Autodesk Inventor part; units mm, degrees
(part 2 of 2)
  line L213 (3.5687, 9.8336) -> (2.9549, 9.8336)
  arc A527 (2.9549, 9.8526) -> (2.9549, 9.8145) centre (2.9549, 9.8336) ccw
  arc A528 (3.5687, 9.8145) -> (3.5687, 9.8526) centre (3.5687, 9.8336) ccw
  arc A529 (2.8321, 9.9563) -> (2.9549, 9.8336) centre (2.9549, 9.9564) ccw
  arc A530 (2.8512, 9.9563) -> (2.8131, 9.9563) centre (2.8321, 9.9563) ccw
  arc A531 (2.9549, 9.8145) -> (2.9549, 9.8526) centre (2.9549, 9.8336) ccw
  line L214 (2.8321, 9.9563) -> (2.8321, 9.9972)
  arc A532 (2.8512, 9.9972) -> (2.8131, 9.9972) centre (2.8321, 9.9972) ccw
  arc A533 (2.8131, 9.9563) -> (2.8512, 9.9563) centre (2.8321, 9.9563) ccw
  line L215 (1.5113, 5.8428) -> (2.2479, 5.8428)
  arc A534 (2.2479, 5.8237) -> (2.2479, 5.8618) centre (2.2479, 5.8427) ccw
  arc A535 (1.5113, 5.8618) -> (1.5113, 5.8237) centre (1.5113, 5.8427) ccw
  line L216 (2.2479, 5.8428) -> (2.2479, 6.0474)
  arc A536 (2.267, 6.0474) -> (2.2288, 6.0474) centre (2.2479, 6.0474) ccw
  arc A537 (2.2288, 5.8428) -> (2.267, 5.8428) centre (2.2479, 5.8428) ccw
  arc A538 (2.2479, 6.0474) -> (1.8387, 6.0474) centre (2.0433, 6.0474) ccw
  arc A539 (2.2288, 6.0474) -> (2.267, 6.0474) centre (2.2479, 6.0474) ccw
  arc A540 (1.8196, 6.0474) -> (1.8577, 6.0474) centre (1.8386, 6.0474) ccw
  line L217 (1.8387, 6.0474) -> (1.8387, 5.8428)
  arc A541 (1.8196, 5.8428) -> (1.8577, 5.8428) centre (1.8386, 5.8428) ccw
  arc A542 (1.8577, 6.0474) -> (1.8196, 6.0474) centre (1.8386, 6.0474) ccw
  line L218 (1.5113, 6.252) -> (1.8387, 6.0883)
  arc A543 (1.8302, 6.0713) -> (1.8472, 6.1053) centre (1.8387, 6.0883) ccw
  arc A544 (1.5198, 6.269) -> (1.5028, 6.235) centre (1.5113, 6.252) ccw
  line L219 (1.5113, 6.9225) -> (1.5113, 6.5951)
  arc A545 (1.4923, 6.5951) -> (1.5304, 6.5951) centre (1.5114, 6.5951) ccw
  arc A546 (1.5304, 6.9225) -> (1.4923, 6.9225) centre (1.5114, 6.9225) ccw
  line L220 (1.5113, 6.5951) -> (2.2479, 6.5951)
  arc A547 (2.2479, 6.5761) -> (2.2479, 6.6142) centre (2.2479, 6.5952) ccw
  arc A548 (1.5113, 6.6142) -> (1.5113, 6.5761) centre (1.5113, 6.5952) ccw
  line L221 (2.2479, 6.5951) -> (2.2479, 6.9225)
  arc A549 (2.267, 6.9225) -> (2.2288, 6.9225) centre (2.2479, 6.9225) ccw
  arc A550 (2.2288, 6.5951) -> (2.267, 6.5951) centre (2.2479, 6.5951) ccw
  line L222 (1.9205, 6.5951) -> (1.9205, 6.8407)
  arc A551 (1.9396, 6.8407) -> (1.9015, 6.8407) centre (1.9205, 6.8407) ccw
  arc A552 (1.9015, 6.5951) -> (1.9396, 6.5951) centre (1.9205, 6.5951) ccw
  line L223 (2.2479, 7.1622) -> (1.5113, 7.4078)
  arc A553 (1.5173, 7.4258) -> (1.5053, 7.3897) centre (1.5113, 7.4078) ccw
  arc A554 (2.2419, 7.1442) -> (2.2539, 7.1803) centre (2.2479, 7.1623) ccw
  arc A555 (1.651, 2.54) -> (1.651, 3.81) centre (1.651, 3.175) ccw
  arc A556 (1.651, 3.81) -> (1.651, 2.54) centre (1.651, 3.175) ccw
  arc A557 (1.651, 1.778) -> (1.651, 0.508) centre (1.651, 1.143) ccw
  arc A558 (1.651, 0.508) -> (1.651, 1.778) centre (1.651, 1.143) ccw
  arc A559 (10.16, 11.938) -> (10.16, 13.208) centre (10.16, 12.573) ccw
  arc A560 (10.16, 13.208) -> (10.16, 11.938) centre (10.16, 12.573) ccw
  line L224 (0.514, 8.885) -> (7.614, 8.885)
  arc A561 (7.614, 8.8342) -> (7.614, 8.9358) centre (7.614, 8.885) ccw
  arc A562 (0.514, 8.9358) -> (0.514, 8.8342) centre (0.514, 8.885) ccw
  line L225 (7.614, 8.885) -> (7.614, 5.585)
  arc A563 (7.5632, 5.585) -> (7.6648, 5.585) centre (7.614, 5.585) ccw
  arc A564 (7.6648, 8.885) -> (7.5632, 8.885) centre (7.614, 8.885) ccw
  line L226 (0.514, 5.585) -> (0.514, 8.885)
  arc A565 (0.5648, 8.885) -> (0.4632, 8.885) centre (0.514, 8.885) ccw
  arc A566 (0.4632, 5.585) -> (0.5648, 5.585) centre (0.514, 5.585) ccw
  line L227 (0.364, 8.935) -> (0.214, 8.935)
  arc A567 (0.214, 8.9604) -> (0.214, 8.9096) centre (0.214, 8.935) ccw
  arc A568 (0.364, 8.9096) -> (0.364, 8.9604) centre (0.364, 8.935) ccw
  line L228 (0.214, 8.935) -> (0.214, 8.635)
  arc A569 (0.1886, 8.635) -> (0.2394, 8.635) centre (0.214, 8.635) ccw
  arc A570 (0.2394, 8.935) -> (0.1886, 8.935) centre (0.214, 8.935) ccw
  line L229 (0.214, 8.635) -> (-0.386, 8.635)
  arc A571 (-0.386, 8.6604) -> (-0.386, 8.6096) centre (-0.386, 8.635) ccw
  arc A572 (0.214, 8.6096) -> (0.214, 8.6604) centre (0.214, 8.635) ccw
  line L230 (-0.386, 8.635) -> (-0.386, 8.435)
  arc A573 (3.683, 2.54) -> (3.683, 3.81) centre (3.683, 3.175) ccw
  arc A574 (3.683, 3.81) -> (3.683, 2.54) centre (3.683, 3.175) ccw
  arc A575 (-0.4114, 8.435) -> (-0.3606, 8.435) centre (-0.386, 8.435) ccw
  arc A576 (-0.3606, 8.635) -> (-0.4114, 8.635) centre (-0.386, 8.635) ccw
  line L231 (-0.386, 8.435) -> (0.214, 8.435)
  arc A577 (0.214, 8.4096) -> (0.214, 8.4604) centre (0.214, 8.435) ccw
  arc A578 (-0.386, 8.4604) -> (-0.386, 8.4096) centre (-0.386, 8.435) ccw
  line L232 (0.214, 8.435) -> (0.214, 7.935)
  arc A579 (0.1886, 7.935) -> (0.2394, 7.935) centre (0.214, 7.935) ccw
  line L233 (0.214, 7.935) -> (0.164, 7.885)
  arc A580 (0.146, 7.903) -> (0.182, 7.867) centre (0.164, 7.885) ccw
  arc A581 (3.683, 0.508) -> (3.683, 1.778) centre (3.683, 1.143) ccw
  arc A582 (3.683, 1.778) -> (3.683, 0.508) centre (3.683, 1.143) ccw
  arc A583 (0.232, 7.917) -> (0.196, 7.953) centre (0.214, 7.935) ccw
  line L234 (0.164, 7.885) -> (-0.386, 7.885)
  arc A584 (-0.386, 7.9104) -> (-0.386, 7.8596) centre (-0.386, 7.885) ccw
  arc A585 (0.164, 7.8596) -> (0.164, 7.9104) centre (0.164, 7.885) ccw
  line L235 (-0.386, 7.885) -> (-0.386, 7.685)
  arc A586 (-0.4114, 7.685) -> (-0.3606, 7.685) centre (-0.386, 7.685) ccw
  arc A587 (-0.3606, 7.885) -> (-0.4114, 7.885) centre (-0.386, 7.885) ccw
  line L236 (-0.386, 7.685) -> (0.364, 7.685)
  arc A588 (0.364, 7.6596) -> (0.364, 7.7104) centre (0.364, 7.685) ccw
  arc A589 (-0.386, 7.7104) -> (-0.386, 7.6596) centre (-0.386, 7.685) ccw
  line L237 (0.364, 7.685) -> (0.364, 8.885)
  arc A590 (0.3894, 8.885) -> (0.3386, 8.885) centre (0.364, 8.885) ccw
  arc A591 (10.16, 9.906) -> (10.16, 11.176) centre (10.16, 10.541) ccw
  arc A592 (10.16, 11.176) -> (10.16, 9.906) centre (10.16, 10.541) ccw
  arc A593 (0.3386, 7.685) -> (0.3894, 7.685) centre (0.364, 7.685) ccw
  arc A594 (0.2394, 8.435) -> (0.1886, 8.435) centre (0.214, 8.435) ccw
  line L238 (1.251, 0.9772) -> (1.251, 1.3088)
  line L239 (1.251, 1.3088) -> (1.4852, 1.5431)
  line L240 (1.4852, 1.5431) -> (1.8168, 1.5431)
  line L241 (1.8168, 1.5431) -> (2.0511, 1.3088)
  line L242 (2.0511, 1.3088) -> (2.0511, 0.9772)
  line L243 (2.0511, 0.9772) -> (1.8168, 0.7429)
  line L244 (1.8168, 0.7429) -> (1.4852, 0.7429)
  line L245 (1.4852, 0.7429) -> (1.251, 0.9772)
  line L246 (1.251, 0.9772) -> (1.251, 1.3088)
  line L247 (1.251, 0.9772) -> (1.251, 1.3088)
  line L248 (1.251, 1.3088) -> (1.4852, 1.5431)
  line L249 (1.4852, 1.5431) -> (1.8168, 1.5431)
  line L250 (1.8168, 1.5431) -> (2.0511, 1.3088)
  line L251 (2.0511, 1.3088) -> (2.0511, 0.9772)
  line L252 (2.0511, 0.9772) -> (1.8168, 0.7429)
  line L253 (1.8168, 0.7429) -> (1.4852, 0.7429)
  line L254 (1.4852, 0.7429) -> (1.251, 0.9772)
  line L255 (1.251, 0.9772) -> (1.251, 1.3088)
  line L256 (9.7599, 10.3752) -> (9.7599, 10.7068)
  line L257 (9.7599, 10.7068) -> (9.9942, 10.9411)
  line L258 (9.9942, 10.9411) -> (10.3258, 10.9411)
  line L259 (10.3258, 10.9411) -> (10.5601, 10.7068)
  line L260 (10.5601, 10.7068) -> (10.5601, 10.3752)
  line L261 (10.5601, 10.3752) -> (10.3258, 10.141)
  line L262 (10.3258, 10.141) -> (9.9942, 10.141)
  line L263 (9.9942, 10.141) -> (9.7599, 10.3752)
  line L264 (9.7599, 10.3752) -> (9.7599, 10.7068)
  line L265 (9.7599, 10.3752) -> (9.7599, 10.7068)
  line L266 (9.7599, 10.7068) -> (9.9942, 10.9411)
  line L267 (9.9942, 10.9411) -> (10.3258, 10.9411)
  line L268 (10.3258, 10.9411) -> (10.5601, 10.7068)
  line L269 (10.5601, 10.7068) -> (10.5601, 10.3752)
  line L270 (10.5601, 10.3752) -> (10.3258, 10.141)
  line L271 (10.3258, 10.141) -> (9.9942, 10.141)
  line L272 (9.9942, 10.141) -> (9.7599, 10.3752)
  line L273 (9.7599, 10.3752) -> (9.7599, 10.7068)
  line L274 (9.7599, 12.4072) -> (9.7599, 12.7388)
  line L275 (9.7599, 12.7388) -> (9.9942, 12.9731)
  line L276 (9.9942, 12.9731) -> (10.3258, 12.9731)
  line L277 (10.3258, 12.9731) -> (10.5601, 12.7388)
  line L278 (10.5601, 12.7388) -> (10.5601, 12.4072)
  line L279 (10.5601, 12.4072) -> (10.3258, 12.173)
  line L280 (10.3258, 12.173) -> (9.9942, 12.173)
  line L281 (9.9942, 12.173) -> (9.7599, 12.4072)
  line L282 (9.7599, 12.4072) -> (9.7599, 12.7388)
  line L283 (9.7599, 12.4072) -> (9.7599, 12.7388)
  line L284 (9.7599, 12.7388) -> (9.9942, 12.9731)
  line L285 (9.9942, 12.9731) -> (10.3258, 12.9731)
  line L286 (10.3258, 12.9731) -> (10.5601, 12.7388)
  line L287 (10.5601, 12.7388) -> (10.5601, 12.4072)
  line L288 (10.5601, 12.4072) -> (10.3258, 12.173)
  line L289 (10.3258, 12.173) -> (9.9942, 12.173)
  line L290 (9.9942, 12.173) -> (9.7599, 12.4072)
  line L291 (9.7599, 12.4072) -> (9.7599, 12.7388)
  line L292 (3.283, 3.0092) -> (3.283, 3.3408)
  line L293 (3.283, 3.3408) -> (3.5172, 3.5751)
  line L294 (3.5172, 3.5751) -> (3.8488, 3.5751)
  line L295 (3.8488, 3.5751) -> (4.0831, 3.3408)
  line L296 (4.0831, 3.3408) -> (4.0831, 3.0092)
  line L297 (4.0831, 3.0092) -> (3.8488, 2.775)
  line L298 (3.8488, 2.775) -> (3.5172, 2.775)
  line L299 (3.5172, 2.775) -> (3.283, 3.0092)
  line L300 (3.283, 3.0092) -> (3.283, 3.3408)
  line L301 (3.283, 3.0092) -> (3.283, 3.3408)
  line L302 (3.283, 3.3408) -> (3.5172, 3.5751)
  line L303 (3.5172, 3.5751) -> (3.8488, 3.5751)
  line L304 (3.8488, 3.5751) -> (4.0831, 3.3408)
  line L305 (4.0831, 3.3408) -> (4.0831, 3.0092)
  line L306 (4.0831, 3.0092) -> (3.8488, 2.775)
  line L307 (3.8488, 2.775) -> (3.5172, 2.775)
  line L308 (3.5172, 2.775) -> (3.283, 3.0092)
  line L309 (3.283, 3.0092) -> (3.283, 3.3408)
  line L310 (3.283, 0.9772) -> (3.283, 1.3088)
  line L311 (3.283, 1.3088) -> (3.5172, 1.5431)
  line L312 (3.5172, 1.5431) -> (3.8488, 1.5431)
  line L313 (3.8488, 1.5431) -> (4.0831, 1.3088)
  line L314 (4.0831, 1.3088) -> (4.0831, 0.9772)
  line L315 (4.0831, 0.9772) -> (3.8488, 0.7429)
  line L316 (3.8488, 0.7429) -> (3.5172, 0.7429)
  line L317 (3.5172, 0.7429) -> (3.283, 0.9772)
  line L318 (3.283, 0.9772) -> (3.283, 1.3088)
  line L319 (3.283, 0.9772) -> (3.283, 1.3088)
  line L320 (3.283, 1.3088) -> (3.5172, 1.5431)
  line L321 (3.5172, 1.5431) -> (3.8488, 1.5431)
  line L322 (3.8488, 1.5431) -> (4.0831, 1.3088)
  line L323 (4.0831, 1.3088) -> (4.0831, 0.9772)
  line L324 (4.0831, 0.9772) -> (3.8488, 0.7429)
  line L325 (3.8488, 0.7429) -> (3.5172, 0.7429)
  line L326 (3.5172, 0.7429) -> (3.283, 0.9772)
  line L327 (3.283, 0.9772) -> (3.283, 1.3088)
  line L328 (6.217, 13.395) -> (6.217, 12.395)
  line L329 (6.217, 12.395) -> (7.217, 12.395)
  line L330 (7.217, 12.395) -> (7.217, 13.395)
  line L331 (7.217, 13.395) -> (6.217, 13.395)
  line L332 (7.067, 13.395) -> (7.067, 12.395)
  line L333 (7.067, 12.395) -> (8.067, 12.395)
  line L334 (8.067, 12.395) -> (8.067, 13.395)
  line L335 (8.067, 13.395) -> (7.067, 13.395)
  line L336 (7.917, 13.395) -> (7.917, 12.395)
  line L337 (7.917, 12.395) -> (8.917, 12.395)
  line L338 (8.917, 12.395) -> (8.917, 13.395)
  line L339 (8.917, 13.395) -> (7.917, 13.395)
  line L340 (7.917, 10.795) -> (7.917, 9.795)
  line L341 (7.917, 9.795) -> (8.917, 9.795)
  line L342 (8.917, 9.795) -> (8.917, 10.795)
  line L343 (8.917, 10.795) -> (7.917, 10.795)
  line L344 (6.217, 10.795) -> (6.217, 9.795)
  line L345 (6.217, 9.795) -> (7.217, 9.795)
  line L346 (7.217, 9.795) -> (7.217, 10.795)
  line L347 (7.217, 10.795) -> (6.217, 10.795)
  line L348 (1.2509, 3.0092) -> (1.2509, 3.3408)
  line L349 (1.2509, 3.3408) -> (1.4852, 3.5751)
  line L350 (1.4852, 3.5751) -> (1.8168, 3.5751)
  line L351 (1.8168, 3.5751) -> (2.0511, 3.3408)
  line L352 (2.0511, 3.3408) -> (2.0511, 3.0092)
  line L353 (2.0511, 3.0092) -> (1.8168, 2.775)
  line L354 (1.8168, 2.775) -> (1.4852, 2.775)
  line L355 (1.4852, 2.775) -> (1.2509, 3.0092)
  line L356 (1.2509, 3.0092) -> (1.2509, 3.3408)
  line L357 (1.2509, 3.0092) -> (1.2509, 3.3408)
  line L358 (1.2509, 3.3408) -> (1.4852, 3.5751)
  line L359 (1.4852, 3.5751) -> (1.8168, 3.5751)
  line L360 (1.8168, 3.5751) -> (2.0511, 3.3408)
  line L361 (2.0511, 3.3408) -> (2.0511, 3.0092)
  line L362 (2.0511, 3.0092) -> (1.8168, 2.775)
  line L363 (1.8168, 2.775) -> (1.4852, 2.775)
  line L364 (1.4852, 2.775) -> (1.2509, 3.0092)
  line L365 (1.2509, 3.0092) -> (1.2509, 3.3408)
  line L366 (2.314, 8.835) -> (3.314, 8.835)
  line L367 (3.314, 8.835) -> (3.314, 9.835)
  line L368 (3.314, 9.835) -> (2.314, 9.835)
  line L369 (2.314, 9.835) -> (2.314, 8.835)
  line L370 (2.814, 8.835) -> (3.814, 8.835)
  line L371 (3.814, 8.835) -> (3.814, 9.835)
  line L372 (3.814, 9.835) -> (2.814, 9.835)
  line L373 (2.814, 9.835) -> (2.814, 8.835)
  line L374 (3.314, 8.835) -> (4.314, 8.835)
  line L375 (4.314, 8.835) -> (4.314, 9.835)
  line L376 (4.314, 9.835) -> (3.314, 9.835)
  line L377 (3.314, 9.835) -> (3.314, 8.835)
  line L378 (3.814, 8.835) -> (4.814, 8.835)
  line L379 (4.814, 8.835) -> (4.814, 9.835)
  line L380 (4.814, 9.835) -> (3.814, 9.835)
  line L381 (3.814, 9.835) -> (3.814, 8.835)
  line L382 (4.314, 8.835) -> (5.314, 8.835)
  line L383 (5.314, 8.835) -> (5.314, 9.835)
  line L384 (5.314, 9.835) -> (4.314, 9.835)
  line L385 (4.314, 9.835) -> (4.314, 8.835)
  line L386 (4.814, 8.835) -> (5.814, 8.835)
  line L387 (5.814, 8.835) -> (5.814, 9.835)
  line L388 (5.814, 9.835) -> (4.814, 9.835)
  line L389 (4.814, 9.835) -> (4.814, 8.835)
  line L390 (-0.136, 7.385) -> (0.864, 7.385)
  line L391 (0.864, 7.385) -> (0.864, 8.385)
  line L392 (0.864, 8.385) -> (-0.136, 8.385)
  line L393 (-0.136, 8.385) -> (-0.136, 7.385)
  line L394 (0.414, 5.86) -> (1.414, 5.86)
  line L395 (1.414, 5.86) -> (1.414, 6.86)
  line L396 (1.414, 6.86) -> (0.414, 6.86)
  line L397 (0.414, 6.86) -> (0.414, 5.86)
  line L398 (6.714, 5.86) -> (7.714, 5.86)
  line L399 (7.714, 5.86) -> (7.714, 6.86)
  line L400 (7.714, 6.86) -> (6.714, 6.86)
  line L401 (6.714, 6.86) -> (6.714, 5.86)
  line L402 (2.314, 8.985) -> (3.314, 8.985)
  line L403 (3.314, 8.985) -> (3.314, 9.985)
  line L404 (3.314, 9.985) -> (2.314, 9.985)
  line L405 (2.314, 9.985) -> (2.314, 8.985)
  line L406 (2.814, 8.985) -> (3.814, 8.985)
  line L407 (3.814, 8.985) -> (3.814, 9.985)
  line L408 (3.814, 9.985) -> (2.814, 9.985)
  line L409 (2.814, 9.985) -> (2.814, 8.985)
  line L410 (3.314, 8.985) -> (4.314, 8.985)
  line L411 (4.314, 8.985) -> (4.314, 9.985)
  line L412 (4.314, 9.985) -> (3.314, 9.985)
  line L413 (3.314, 9.985) -> (3.314, 8.985)
  line L414 (3.814, 8.985) -> (4.814, 8.985)
  line L415 (4.814, 8.985) -> (4.814, 9.985)
  line L416 (4.814, 9.985) -> (3.814, 9.985)
  line L417 (3.814, 9.985) -> (3.814, 8.985)
  line L418 (4.314, 8.985) -> (5.314, 8.985)
  line L419 (5.314, 8.985) -> (5.314, 9.985)
  line L420 (5.314, 9.985) -> (4.314, 9.985)
  line L421 (4.314, 9.985) -> (4.314, 8.985)
  line L422 (4.814, 8.985) -> (5.814, 8.985)
  line L423 (5.814, 8.985) -> (5.814, 9.985)
  line L424 (5.814, 9.985) -> (4.814, 9.985)
  line L425 (4.814, 9.985) -> (4.814, 8.985)
  line L426 (11.43, 9.398) -> (11.43, 12.9549)
  point P0 (0, 0)
  point P1 (4.064, 6.985)
  constraints: 1190 point on circle, 854 end point, 595 centre point, 1 vertical
sketch "Sketch2" plane through (0, 0, 0) normal (0, 1, 0) x (-1, 0, 0)
  line L0 (10.6689, 13.716) -> (6.096, 13.716)
  line L1 (6.096, 13.716) -> (6.096, 12.446)
  line L2 (6.096, 12.446) -> (3.81, 12.446)
  line L3 (3.81, 12.446) -> (2.286, 10.922)
  line L4 (2.286, 10.922) -> (2.286, 9.144)
  line L5 (2.286, 9.144) -> (0.127, 9.144)
  line L6 (0.127, 9.144) -> (0.127, 1.143)
  line L7 (0.127, 1.143) -> (1.27, 0)
  line L8 (1.27, 0) -> (4.572, 0)
  line L9 (4.572, 0) -> (5.334, 0.762)
  line L10 (5.334, 0.762) -> (5.334, 5.588)
  line L11 (5.334, 5.588) -> (7.62, 5.588)
  line L12 (7.62, 5.588) -> (7.62, 8.89)
  line L13 (7.62, 8.89) -> (8.128, 9.398)
  line L14 (8.128, 9.398) -> (11.43, 9.398)
  line L15 (11.43, 9.398) -> (11.43, 12.9549)
  line L16 (11.43, 12.9549) -> (10.6689, 13.716)
  point P0 (5.334, 0.762)
  constraints: 34 end point, 8 perpendicular, 6 parallel, 1 coincident, 1 horizontal
extrude "Extrusion1" add sketch "Sketch2" along normal blind 0.6
sketch "Sketch3" plane through (0, 0, 0) normal (0, -1, 0) x (1, 0, 0)
  line L0 (0.286, 3.385) -> (-8.414, 3.385) projected
  line L1 (-0.514, 8.885) -> (-7.614, 8.885)
  line L2 (-7.614, 8.885) -> (-7.614, 5.585)
  line L3 (-7.614, 5.585) -> (-7.614, 3.385)
  line L4 (-0.514, 3.385) -> (-0.514, 8.885)
  point P0 (0, 0)
  point P1 (-0.514, 5.585)
  constraints: 8 end point, 4 point on line, 1 horizontal, 1 perpendicular
extrude "Extrusion2" add sketch "Sketch3" against normal blind 2 from surface at -0.6 separate body
body "Solid1"
body "Solid2"
